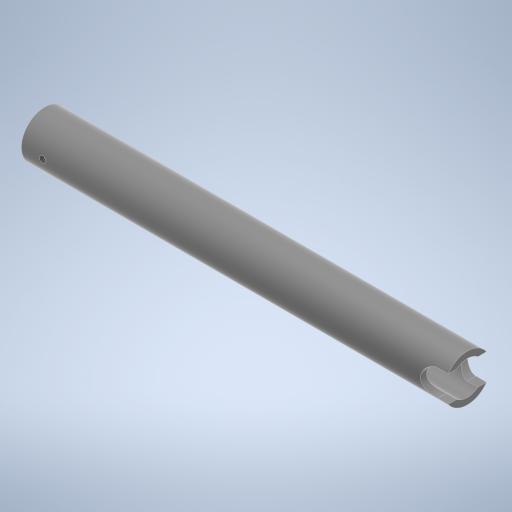
# Autodesk Inventor part: vp16_200
Saved by Autodesk Inventor 2024 (Build 280153000, 153)
## iProperties
Created: 2024-10-07
Part Number: vp16_200
Material: PVC 配管
Document SubType Name: Modeling
Designer: 1412z
Density: 1.4 g/cm^3
Appearance: 滑らか - 濃い灰色
Author: 1412z
Autodesk Inventor part; units mm, degrees
ref_plane "YZ Plane" through (0, 0, 0) normal (1, 0, 0) x (0, 1, 0)
ref_plane "XZ Plane" through (0, 0, 0) normal (0, 1, 0) x (-1, 0, 0)
ref_plane "XY Plane" through (0, 0, 0) normal (0, 0, 1) x (1, 0, 0)
sketch "スケッチ1" plane through (0, 0, 0) normal (1, 0, 0) x (0, 1, 0)
  circle A0 centre (0, 0) radius 11
  circle A1 centre (0, 0) radius 8
  dimension "d0" = 22
  dimension "d1" = 16
  constraints: 2 centre point, 2 coincident
  measures "d0" diameter of A0
  measures "d1" diameter of A1
extrude "押し出し1" add sketch "スケッチ1" against normal blind 200
sketch "スケッチ2" plane through (0, 0, 0) normal (0, 0, 1) x (1, 0, 0)
  line L0 (0, 0) -> (0, 6.25)
  line L1 (0, -11) -> (0, 11) projected
  line L2 (0, 0) -> (0, -6.25)
  line L3 (0, -6.25) -> (-5, -6.25)
  line L4 (-5, -6.25) -> (-5, 6.25)
  line L5 (-5, 6.25) -> (0, 6.25)
  dimension "d4" = 6.25
  dimension "d5" = 6.25
  dimension "d6" = 5
  constraints: 10 end point, 2 perpendicular, 2 point on line, 1 horizontal
  measures "d4" distance of L0.start L0.end
  measures "d5" distance of L0.start L2.end
  measures "d6" distance of L2.end L3.end
extrude "押し出し2" cut sketch "スケッチ2" along normal mid plane 200
sketch "スケッチ3" plane through (0, 0, 0) normal (0, 0, 1) x (1, 0, 0)
  line L0 (-5, -6.25) -> (-5, 6.25) projected
  circle A0 centre (-5, 0) radius 6.25
  point P0 (0, 0)
  constraints: 1 midpoint, 3 other
extrude "押し出し3" cut sketch "スケッチ3" along normal mid plane 200 contours A0 L0 picked at (-7.0681, 0.2511)
sketch "スケッチ4" plane through (0, 0, 0) normal (0, 0, 1) x (1, 0, 0)
  circle A0 centre (-190, 0) radius 1.5
  point P0 (0, 0)
  dimension "d11" = 3
  constraints: 1 centre point
  measures "d11" diameter of A0
extrude "押し出し4" cut sketch "スケッチ4" along normal mid plane 200
thread "ねじ1" size "M3x0.5" class "6H" standard "ANSI Metric M Profile" full length
thread "ねじ2" size "M3x0.5" class "6H" standard "ANSI Metric M Profile" full length
